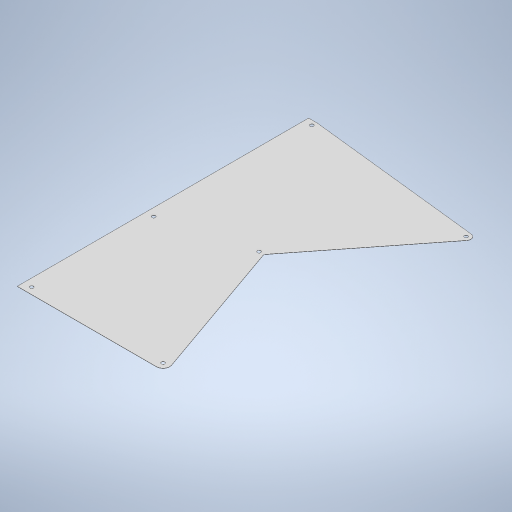
# Autodesk Inventor part: base_main_pcb_full_itr3
Saved by Autodesk Inventor 2024 (Build 280153000, 153)
## iProperties
Created: 2026-03-21
Part Number: base_main_pcb_full_itr3
Material: Generic
Document SubType Name: Modeling
Designer: schar
Density: 1 g/cm^3
Appearance: Default
Author: schar
Autodesk Inventor part; units mm, degrees
ref_plane "YZ Plane" through (0, 0, 0) normal (1, 0, 0) x (0, 1, 0)
ref_plane "XZ Plane" through (0, 0, 0) normal (0, 1, 0) x (-1, 0, 0)
ref_plane "XY Plane" through (0, 0, 0) normal (0, 0, 1) x (1, 0, 0)
ref_plane "Work Plane1" through (-205, 2, 0) normal (0, 1, 0) x (1, 0, 0)
sketch "Sketch2" plane through (-205, 2, 0) normal (0, 1, 0) x (1, 0, 0)
  circle A0 centre (86.5, -146.525) radius 1.675 projected
  circle A1 centre (86.5, -146.525) radius 1.675
  circle A2 centre (86.5, -146.525) radius 4.5
  circle A3 centre (172.5, -35.525) radius 1.675 projected
  circle A4 centre (172.5, -35.525) radius 1.675
  circle A5 centre (172.5, -35.525) radius 4.5
  circle A6 centre (132.5, -283.785) radius 1.675 projected
  circle A7 centre (132.5, -283.785) radius 6.215
  line L0 (0, -290) -> (155, -290) projected
  circle A8 centre (7.5, -283.785) radius 1.675 projected
  circle A9 centre (7.5, -283.785) radius 4.5
  circle A10 centre (7.5, -167.775) radius 1.675 projected
  circle A11 centre (7.5, -167.775) radius 4.5
  circle A12 centre (7.5, -17.325) radius 1.675 projected
  circle A13 centre (7.5, -17.325) radius 4.5
  line L1 (0, -290) -> (132.5, -290)
  line L2 (91, -146.525) -> (138.3655, -281.7302)
  line L3 (91, -146.525) -> (176.0383, -38.3054)
  line L4 (172.5, -31.025) -> (7.9941, -12.8522)
  line L5 (7.9941, -12.8522) -> (0, -12.8522)
  line L6 (0, -12.8522) -> (0, -290)
  point P0 (205, 0)
  dimension "d3" = 9
  dimension "d7" = 9
  dimension "d4" = 9
  dimension "d5" = 9
  dimension "d6" = 9
  constraints: 12 end point, 8 coincident, 6 centre point, 4 point on circle, 3 tangent, 1 horizontal, 1 horizontal alignment, 1 perpendicular, 1 point on line, 6 other
  measures "d4" diameter of A5
  measures "d5" diameter of A9
  measures "d6" diameter of A11
extrude "Extrusion1" add sketch "Sketch2" along normal blind 0.2 contours A2 | L2 A7 L0 L6 L5 A13 L4 A5 L3 | A7 | A5 | A13 L5 | A9 | A11 picked at (10.9979, -16.8298)
body "Solid2"
